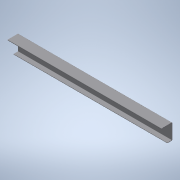
# Autodesk Inventor part: SP38V1 Cobertor Freno
Saved by Autodesk Inventor 2021.2 (Build 252289000, 289)
## iProperties
Created: 2026-08-21
Part Number: SP38V1 Cobertor Freno
Material: Generic
Document SubType Name: Sheet Metal
Designer: nelso
Density: 1 g/cm^3
Sheet Metal Rule: Default_mm
Appearance: Default
Author: nelso
Autodesk Inventor part; units mm, degrees
ref_plane "YZ Plane" through (0, 0, 0) normal (1, 0, 0) x (0, 1, 0)
ref_plane "XZ Plane" through (0, 0, 0) normal (0, 1, 0) x (-1, 0, 0)
ref_plane "XY Plane" through (0, 0, 0) normal (0, 0, 1) x (1, 0, 0)
sketch "Sketch1" plane through (0, 0, 0) normal (0, 1, 0) x (-1, 0, 0)
  line L0 (395, 40.5) -> (-395, 40.5)
  line L1 (-395, 40.5) -> (-395, -40.5)
  line L2 (-395, -40.5) -> (395, -40.5)
  line L3 (395, -40.5) -> (395, 40.5)
  line L4 (395, 40.5) -> (-395, -40.5) construction
  line L5 (-395, 40.5) -> (395, -40.5) construction
  point P0 (0, 0)
  dimension "d0" = 790
  dimension "d1" = 81
  measures "d0" distance of L2.end L1.end
  measures "d1" distance of L1.end L0.end
extrude "Plate1" add sketch "Sketch1" along normal blind 2.1
sketch "Sketch2" plane through (-395, 2.1, -38.4) normal (0, 0, -1) x (-1, 0, 0)
  line L0 (-790, 0) -> (0, 0)
  line L1 (0, 0) -> (0, 25)
  line L2 (0, 25) -> (-790, 25)
  line L3 (-790, 25) -> (-790, 0)
  constraints: 6 end point, 1 horizontal, 1 perpendicular, 1 vertical
edge flange "Flange1" height 25 angle 90 thickness 2.1 bend radius 1.512 thickness toward (0, 0, -1) relief straight relief width 2.1 relief depth 1.05 edges at (0, 2.1, -40.5) wall of the first edge with corners at (395, 2.1, -38.4) (-395, 2.1, -38.4) (-395, -22.9, -38.4) (395, -22.9, -38.4)
bend "Bend1"
corner "Corner1"
sketch "Sketch3" plane through (395, 2.1, 38.4) normal (0, 0, 1) x (1, 0, 0)
  line L0 (-790, 0) -> (0, 0)
  line L1 (0, 0) -> (0, 54.6)
  line L2 (0, 54.6) -> (-790, 54.6)
  line L3 (-790, 54.6) -> (-790, 0)
  constraints: 6 end point, 1 horizontal, 1 perpendicular, 1 vertical
edge flange "Flange2" height 54.6 angle 90 thickness 2.1 bend radius 1.512 thickness toward (0, 0, 1) relief straight relief width 2.1 relief depth 1.05 edges at (0, 2.1, 40.5) wall of the first edge with corners at (-395, 2.1, 38.4) (395, 2.1, 38.4) (395, -52.5, 38.4) (-395, -52.5, 38.4)
bend "Bend2"
corner "Corner2"
sketch "Sketch4" plane through (395, -49.875, 38.4) normal (1, 0, 0) x (0, 1, 0)
  line L0 (0, 2.1) -> (0, 0)
  arc A0 (0, 0) -> (0, -1.05) centre (0, -0.525) ccw
  line L1 (0, -1.05) -> (5.775, -1.05)
  line L2 (5.775, -1.05) -> (5.775, -3.15)
  line L3 (5.775, -3.15) -> (0, -3.15)
  arc A1 (0, 2.1) -> (0, -3.15) centre (0, -0.525) ccw
  constraints: 8 end point, 4 point on circle
hem "Hem1" sketch "Sketch4" thickness 2.1 along (-1, 0, 0) edges at (0, -52.5, 38.4)
fillet "Corner Round1" radius 2 4 edges at (395, -22.9, -39.45) (395, -44.1, 36.3) (-395, -22.9, -39.45) (-395, -44.1, 36.3)
equation "\"d2\" = Thickness"
equation "\"d23\" = BendReliefWidth"
equation "\"d24\" = BendReliefDepth"
equation "\"d25\" = MinimumRemnant"
equation "\"d26\" = TransitionRadius"
equation "\"d27\" = 4 * Thickness"
equation "\"d28\" = 0.5 * Thickness"
equation "\"d29\" = 0.5 * d28"
equation "\"d3\" = BendReliefWidth"
equation "\"d4\" = BendReliefDepth"
equation "\"d5\" = MinimumRemnant"
equation "\"d6\" = TransitionRadius"
equation "\"d9\" = BendRadius"
equation "\"d10\" = CornerReliefSize"
equation "\"d11\" = GapSize"
equation "\"d12\" = JacobiRadiusSize"
equation "\"d13\" = BendReliefWidth"
equation "\"d14\" = BendReliefDepth"
equation "\"d15\" = MinimumRemnant"
equation "\"d16\" = TransitionRadius"
equation "\"d19\" = BendRadius"
equation "\"d20\" = CornerReliefSize"
equation "\"d21\" = GapSize"
equation "\"d22\" = JacobiRadiusSize"
equation "\"BendReliefWidth\" = Thickness"
equation "\"BendReliefDepth\" = 0.5 * Thickness"
equation "\"CornerReliefSize\" = 4 * Thickness"
equation "\"MinimumRemnant\" = 2 * Thickness"
equation "\"TransitionRadius\" = BendRadius"
equation "\"JacobiRadiusSize\" = BendRadius"
equation "\"GapSize\" = Thickness"
equation "\"Thickness\" = 2.1"
equation "\"BendRadius\" = 1.512"
body "Solid1"
